Autodesk Inventor part; units mm, degrees
(part 2 of 2)
  arc A502 (56.515, 152.1333) -> (56.515, 152.2095) centre (56.515, 152.1714) ccw
  arc A503 (56.515, 156.4513) -> (56.515, 156.5275) centre (56.515, 156.4894) ccw
  arc A504 (46.355, 156.5275) -> (46.355, 156.4513) centre (46.355, 156.4894) ccw
  line L229 (42.335407, 147.261346) -> (42.335407, 160.034298)
  line L230 (57.023, 156.3624) -> (56.515, 156.4894)
  arc A505 (46.3169, 150.7744) -> (46.3931, 150.7744) centre (46.355, 150.7744) ccw
  arc A506 (69.455, 156.8583) -> (69.455, 156.9218) centre (69.455, 156.89005) ccw
  line L231 (69.455, 156.89) -> (70.725, 156.89)
  arc A507 (69.455, 155.5883) -> (69.455, 155.6517) centre (69.455, 155.62) ccw
  arc A508 (69.4232, 155.62) -> (69.4868, 155.62) centre (69.455, 155.62) ccw
  line L232 (69.455, 155.62) -> (69.455, 156.89)
  arc A509 (69.455, 156.9218) -> (69.455, 156.8583) centre (69.455, 156.89005) ccw
  arc A510 (69.4868, 156.89) -> (69.4232, 156.89) centre (69.455, 156.89) ccw
  line L233 (70.725, 156.89) -> (70.725, 151.81)
  arc A511 (70.725, 156.8583) -> (70.725, 156.9218) centre (70.725, 156.89005) ccw
  arc A512 (70.7568, 156.89) -> (70.6933, 156.89) centre (70.72505, 156.89) ccw
  arc A513 (60.5968, 156.89) -> (60.5333, 156.89) centre (60.56505, 156.89) ccw
  line L234 (60.565, 156.89) -> (61.835, 156.89)
  arc A514 (60.565, 156.9218) -> (60.565, 156.8583) centre (60.565, 156.89005) ccw
  arc A515 (68.185, 153.9) -> (68.185, 154.8) centre (68.185, 154.35) ccw
  arc A516 (68.185, 153.9) -> (68.185, 154.8) centre (68.185, 154.35) ccw
  arc A517 (68.185, 154.8) -> (68.185, 153.9) centre (68.185, 154.35) ccw
  arc A518 (68.185, 154.8) -> (68.185, 153.9) centre (68.185, 154.35) ccw
  arc A519 (65.645, 154.8) -> (65.645, 153.9) centre (65.645, 154.35) ccw
  arc A520 (65.645, 154.8) -> (65.645, 153.9) centre (65.645, 154.35) ccw
  arc A521 (61.835, 156.8583) -> (61.835, 156.9218) centre (61.835, 156.89005) ccw
  arc A522 (61.835, 156.9218) -> (61.835, 156.8583) centre (61.835, 156.89005) ccw
  line L235 (61.835, 156.89) -> (61.835, 155.62)
  arc A523 (61.8032, 155.62) -> (61.8668, 155.62) centre (61.835, 155.62) ccw
  arc A524 (61.8668, 156.89) -> (61.8032, 156.89) centre (61.835, 156.89) ccw
  arc A525 (61.835, 155.6517) -> (61.835, 155.5883) centre (61.835, 155.62) ccw
  arc A526 (73.999457, 167.822801) -> (56, 167.7239) centre (65, 167.7239) ccw
  line L236 (51.935, 154.8304) -> (50.935, 154.8304)
  line L237 (48.9204, 153.3398) -> (48.9204, 155.321)
  line L238 (48.9204, 153.3398) -> (48.9204, 155.321)
  line L239 (50.935, 154.8304) -> (50.935, 153.8304)
  line L240 (50.935, 153.8304) -> (51.935, 153.8304)
  arc A527 (54.4449, 155.321) -> (53.4543, 155.321) centre (53.9496, 155.321) ccw
  arc A528 (54.4449, 155.321) -> (53.4543, 155.321) centre (53.9496, 155.321) ccw
  line L241 (53.9496, 153.3398) -> (53.9496, 155.321)
  line L242 (53.9496, 153.3398) -> (53.9496, 155.321)
  line L243 (51.935, 153.8304) -> (51.935, 154.8304)
  arc A529 (53.4543, 153.3398) -> (54.4449, 153.3398) centre (53.9496, 153.3398) ccw
  arc A530 (48.4251, 153.3398) -> (49.4157, 153.3398) centre (48.9204, 153.3398) ccw
  arc A531 (48.4251, 153.3398) -> (49.4157, 153.3398) centre (48.9204, 153.3398) ccw
  arc A532 (53.4543, 153.3398) -> (54.4449, 153.3398) centre (53.9496, 153.3398) ccw
  line L244 (60.565, 151.81) -> (60.565, 156.89)
  arc A533 (60.565, 151.8417) -> (60.565, 151.7783) centre (60.565, 151.81) ccw
  arc A534 (60.5333, 151.81) -> (60.5968, 151.81) centre (60.56505, 151.81) ccw
  line L245 (61.835, 156.89) -> (69.455, 156.89)
  line L246 (61.835, 155.62) -> (69.455, 155.62)
  line L247 (70.725, 151.81) -> (60.565, 151.81)
  arc A535 (70.725, 151.7783) -> (70.725, 151.8417) centre (70.725, 151.81) ccw
  arc A536 (70.6933, 151.81) -> (70.7568, 151.81) centre (70.72505, 151.81) ccw
  line L248 (74.3631, 147.261346) -> (42.335407, 147.261346)
  arc A537 (49.4157, 155.321) -> (48.4251, 155.321) centre (48.9204, 155.321) ccw
  arc A538 (49.4157, 155.321) -> (48.4251, 155.321) centre (48.9204, 155.321) ccw
  line L249 (42.335407, 160.034298) -> (53.975, 160.034298)
  line L250 (74.099451, 167.7239) -> (74.3631, 167.7239)
  line L251 (74.3631, 167.7239) -> (74.3631, 160.034298)
  line L252 (56, 167.7239) -> (55.975, 167.7239)
  line L253 (55.975, 167.7239) -> (55.975, 162.034298)
  arc A539 (73.999457, 167.822801) -> (74.099451, 167.7239) centre (74.099451, 167.8239) ccw
  arc A540 (53.975, 160.034298) -> (55.975, 162.034298) centre (53.975, 162.034298) ccw
  point P0 (0, 0)
  dimension "d4" = 2
  constraints: 1064 point on circle, 541 centre point, 508 end point, 10 coincident, 10 parallel, 6 horizontal, 6 perpendicular, 4 concentric, 4 tangent
  measures "d4" radius of A540
sketch "スケッチ2" plane through (0, 0, 0) normal (0, 0, 1) x (1, 0, 0)
  point P0 (0, 0)
sketch "スケッチ1 outline for 押し出し3" plane through (0, 0, 0) normal (0, 0, 1) x (1, 0, 0)
  line L0 (-10.0002, 0) -> (140.0002, 0)
  line L1 (-10.0002, 194.7239) -> (-10.0002, 0)
  line L2 (140.0002, 0) -> (140.0002, 194.7239)
  line L3 (140.0002, 194.7239) -> (-10.0002, 194.7239)
  circle A0 centre (38, 8) radius 2
  line L4 (28.37271, 25.87255) -> (28.37271, 38.147158)
  line L5 (43.54174, 25.87255) -> (28.37271, 25.87255)
  line L6 (43.54174, 38.147158) -> (43.54174, 25.87255)
  line L7 (28.37271, 38.147158) -> (43.54174, 38.147158)
  circle A1 centre (52, 8) radius 2
  circle A2 centre (78, 8) radius 2
  line L8 (44.73875, 24.202729) -> (44.73875, 33.8709)
  line L9 (94, 24.202729) -> (44.73875, 24.202729)
  line L10 (94, 33.8709) -> (94, 24.202729)
  line L11 (44.73875, 33.8709) -> (94, 33.8709)
  circle A3 centre (92, 8) radius 2
  circle A4 centre (38, 186.7239) radius 2
  arc A5 (74.099451, 167.7239) -> (73.999457, 167.822801) centre (74.099451, 167.8239) cw
  arc A6 (73.999457, 167.822801) -> (56, 167.7239) centre (65, 167.7239) ccw
  line L12 (56, 167.7239) -> (55.975, 167.7239)
  line L13 (55.975, 167.7239) -> (55.975, 162.034298)
  arc A7 (55.975, 162.034298) -> (53.975, 160.034298) centre (53.975, 162.034298) cw
  line L14 (53.975, 160.034298) -> (42.335407, 160.034298)
  line L15 (42.335407, 160.034298) -> (42.335407, 147.261346)
  line L16 (42.335407, 147.261346) -> (74.3631, 147.261346)
  line L17 (74.3631, 147.261346) -> (74.3631, 160.034298)
  line L18 (74.3631, 160.034298) -> (74.3631, 167.7239)
  line L19 (74.3631, 167.7239) -> (74.099451, 167.7239)
  circle A8 centre (52, 186.7239) radius 2
  circle A9 centre (65, 97.362) radius 9
  circle A10 centre (78, 186.7239) radius 2
  line L20 (78, 168.379005) -> (78, 180.99093)
  line L21 (100.51742, 168.379005) -> (78, 168.379005)
  line L22 (100.51742, 180.99093) -> (100.51742, 168.379005)
  line L23 (78, 180.99093) -> (100.51742, 180.99093)
  circle A11 centre (92, 186.7239) radius 2
extrude "押し出し3" add sketch "スケッチ1 outline for 押し出し3" along normal blind 2
